Autodesk Fusion 360 part; units mm, degrees
(part 4 of 4)
sketch "Sketch4" plane through (0, 1.5, 0) normal (0, 1, 0) x (-1, 0, 0)
  line L0 (-160.2375, -0.05) -> (-160.2375, 50.95)
  line L1 (-160.2375, 50.95) -> (-169.7625, 50.95)
  line L2 (-169.7625, 50.95) -> (-169.7625, 70)
  line L3 (-169.7625, 70) -> (-155.475, 70)
  line L4 (-155.475, 70) -> (-155.475, 89.05)
  line L5 (-155.475, 89.05) -> (-165, 89.05)
  line L6 (-162.7625, 24.1125) -> (-162.7625, 11.1125)
  line L7 (-153.7375, 53.475) -> (-166.7375, 53.475)
  line L8 (-167.2375, 53.975) -> (-167.2375, 66.975)
  line L9 (-158.5, 72.525) -> (-171.5, 72.525)
  line L10 (-158, 86.025) -> (-158, 73.025)
  line L11 (-148.975, 91.575) -> (-161.975, 91.575)
  line L12 (-162.475, 92.075) -> (-162.475, 105.075)
  line L13 (-165, 89.05) -> (-165, 140)
  line L14 (-160.2375, -0.05) -> (0, 0)
  line L15 (-165, 140) -> (0, 140)
  line L16 (0, 140) -> (0, 0)
  dimension "d20" = 2.525
  dimension "d21" = 2.525
  dimension "d22" = 2.525
  dimension "d23" = 2.525
  dimension "d24" = 2.525
  dimension "d25" = 2.525
  dimension "d27" = 2.525
  constraint perpendicular L1 L2
  constraint perpendicular L1 L4
  constraint perpendicular L5 L13
  constraint coincident L14.end L16.end
  constraint perpendicular L13 L15
  constraint parallel L13 L16
  measures "d20" distance of L0 L6
  measures "d21" distance of L1 L7
  measures "d22" distance of L2 L8
  measures "d23" distance of L3 L9
  measures "d24" distance of L4 L10
  measures "d25" distance of L5 L11
  measures "d27" distance of L12 L13
extrude "Extrude4" cut sketch "Sketch4" against normal blind 1.5 keep common part bodies 1
extrude "Extrude1'" add sketch "Sketch3" along normal blind 1.5 separate body makes body 2 in component "Component"
copy_body "Body->Comp1" bodies 1 removing the originals makes body 3 in component "Component'"
extrude "Extrude2'" cut 1 faces at (111.6625, 1.5, 118.6083) along direction (0, 1, 0) blind 8 on bodies 3 bodies 2 in component "Component"
fillet "Fillet1'" radius 0.5 18 edges at (246, 3, 140) (329.1213, 3, 139.1213) (330, 3, 103.7375) (329.1213, 3, 68.3537) (312.2938, 3, 67.475) (295.4662, 3, 66.5963) (294.5875, 3, 33.7375) (293.7088, 3, 0.8787) (225.9125, 3, 0) (246, 1.5, 140) (329.1213, 1.5, 139.1213) (330, 1.5, 103.7375) (329.1213, 1.5, 68.3537) (312.2938, 1.5, 67.475) (295.4662, 1.5, 66.5963) (294.5875, 1.5, 33.7375) (293.7088, 1.5, 0.8787) (225.9125, 1.5, 0) on bodies 2 in component "Component"
fillet "Fillet1''" radius 0.5 10 edges at (81.6188, 1.5, 0) (0.8787, 1.5, 0.8787) (0, 1.5, 70) (0.8787, 1.5, 139.1213) (84, 1.5, 140) (84, 0, 140) (0.8787, 0, 139.1213) (0, 0, 70) (0.8787, 0, 0.8787) (81.6188, 0, 0) on bodies 3 in component "Component'"
component "Component" placed x (1, 0, 0) y (0, 1, 0) z (0, 0, 1) at (0, 0, 0)
component "Component'" placed x (1, 0, 0) y (0, 1, 0) z (0, 0, 1) at (0, 0, 0)
equation "d20 = ( 5.05 / 2 ) * 1 mm"
equation "d21 = ( 5.05 / 2 ) * 1 mm"
equation "d22 = ( 5.05 / 2 ) * 1 mm"
equation "d24 = ( 5.05 / 2 ) * 1 mm"
equation "d25 = ( 5.05 / 2 ) * 1 mm"
equation "d27 = ( 5.05 / 2 ) * 1 mm"
